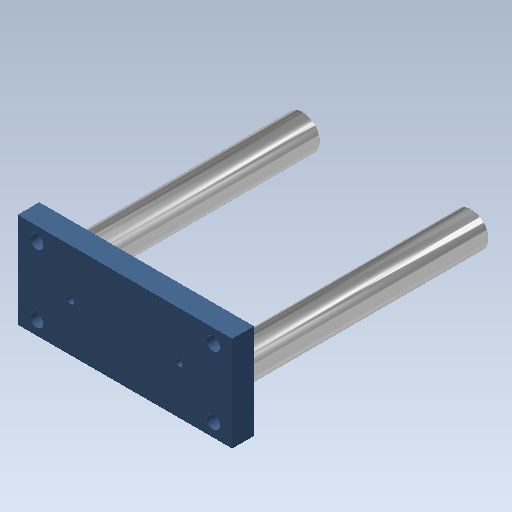
# Autodesk Inventor part: ADSK-MH-10030
Saved by Autodesk Inventor 2020.2 (Build 242310000, 310)
## iProperties
Created: 2008-03-10
Part Number: ADSK-MH-10030
Document SubType Name: Modeling
Designer: R.O'mahony
Density: 2.71 g/cm^3
Mass: 935.152 g
Surface Area: 590.255 cm^2
Volume: 345.074 cm^3
Material: Aluminum 6061
Appearance: Chrome - Polished
Description: Pneumatic Piston
Engineer: Demir Ali
Checked By: Demir Ali
Company: Autodesk Ltd
Author: R.O'mahony
Keywords: Roller Conveyor
Revision Number: A
Autodesk Inventor part; units mm, degrees
ref_plane "YZ Plane" through (0, 0, 0) normal (1, 0, 0) x (0, 1, 0)
ref_plane "XZ Plane" through (0, 0, 0) normal (0, 1, 0) x (-1, 0, 0)
ref_plane "XY Plane" through (0, 0, 0) normal (0, 0, 1) x (1, 0, 0)
sketch "Sketch1" plane through (0, 0, 0) normal (0, 0, 1) x (1, 0, 0)
  line L0 (2448.8434, -559.2477) -> (2606.8434, -559.2477)
  line L1 (2606.8434, -489.2477) -> (2448.8434, -489.2477)
  line L2 (2448.8434, -489.2477) -> (2448.8434, -559.2477)
  circle A0 centre (2462.8434, -549.2477) radius 5
  arc A1 (2487.8434, -526.7477) -> (2487.8434, -521.7477) centre (2487.8434, -524.2477) ccw
  arc A2 (2487.8434, -521.7477) -> (2487.8434, -526.7477) centre (2487.8434, -524.2477) ccw
  line L3 (2487.3434, -526.7477) -> (2488.3434, -526.7477)
  line L4 (2488.3434, -521.7477) -> (2487.3434, -521.7477)
  circle A3 centre (2462.8434, -499.2477) radius 5
  line L5 (2606.8434, -559.2477) -> (2606.8434, -489.2477)
  circle A4 centre (2592.8434, -549.2477) radius 5
  circle A5 centre (2592.8434, -499.2477) radius 5
  circle A6 centre (2567.8434, -524.2477) radius 2.5
  point P0 (0, 0)
  constraints: 12 end point, 7 centre point, 4 point on circle, 2 midpoint
extrude "Extrusion1" add sketch "Sketch1" along normal blind 16
sketch "Sketch2" plane through (0, 0, 0) normal (0, 0, -1) x (-1, 0, 0)
  circle A0 centre (-2487.8434, -524.2477) radius 2.5
  circle A1 centre (-2567.8434, -524.2477) radius 2.5
  circle A2 centre (-2589.8434, -524.2477) radius 12.5
  circle A3 centre (-2465.8434, -524.2477) radius 12.5
  line L0 (-2527.8434, -524.2477) -> (-2527.8434, -513.4708)
  point P0 (0, 0)
  dimension "d2" = 25
  dimension "d3" = 25
  dimension "d8" = 124
  dimension "d9" = 62
  constraints: 4 centre point, 2 end point
  measures "d2" diameter of A2
  measures "d3" diameter of A3
  measures "d8" distance of A3.centre A2.centre
  measures "d9" distance from line of A2.centre L0
extrude "Extrusion2" add sketch "Sketch2" along normal blind 177 contours A2 | A3
body "Solid1"
